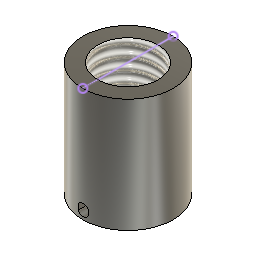
homemaderotoforgetoolholder v5 (Autodesk Fusion 360 archive; units mm, degrees)
design "homemaderotoforgetoolholder" references "autodesk 3ax table y head xz"
Autodesk Fusion 360 part; units mm, degrees
sketch "Sketch1" plane through (0, 0, 0) normal (0, 0, 1) x (1, 0, 0)
  circle A0 centre (0, 0) radius 3.175
  dimension "d1" = 6.35
  constraint coincident A0.centre origin
  measures "d1" diameter of A0
extrude "Extrude1" add sketch "Sketch1" along normal blind 8
sketch "Sketch2" plane through (0, 0, 8) normal (0, 0, 1) x (-1, 0, 0)
  circle A0 centre (0, 0) radius 3.175
  circle A1 centre (0, 0) radius 2
  constraint coincident A0.centre A1.centre
hole "Hole1" at (0, 0, 8) direction (0, 0, -1) diameter 4.234 depth 8 tip angle 180
thread "Thread1" "ISO Metric profile 5.0 M5x0.8 6H" major diameter 5.12 minor diameter 4.234 pitch 0.8 angle 60 resizes the face on face at (0.2108, -2.1065, 5.3333) from (0, 0, 8) to (0, 0, 1.5)
sketch "Sketch4" plane through (0, 0, 0) normal (1, 0, 0) x (0, 1, 0)
  line L0 (3.175, 8) -> (-3.175, 8)
sketch "Sketch5" plane through (0, 0, 0) normal (0, 0, -1) x (1, 0, 0)
  circle A0 centre (0, 0) radius 2.117
  circle A1 centre (0, 0) radius 3.175
  circle A2 centre (0, 0) radius 3.5
  circle A3 centre (0, 0) radius 2.117
  circle A4 centre (0, 0) radius 1.1
  dimension "d17" = 7
  dimension "d18" = 4.234
  dimension "d19" = 2.2
  constraint coincident A0.centre A1.centre
  constraint concentric A2 A3
  measures "d17" diameter of A2
  measures "d18" diameter of A3
  measures "d19" diameter of A4
extrude "Extrude3" add sketch "Sketch5" against normal blind 1.2 contours A0 A3
sketch "Sketch3" plane through (0, 0, 0) normal (0, 1, 0) x (1, 0, 0)
  line L0 (-0.5, -0.1) -> (0.5, -0.1)
  line L1 (0.5, -0.1) -> (0.5, -1.1)
  line L2 (0.5, -1.1) -> (-0.5, -1.1)
  line L3 (-0.5, -1.1) -> (-0.5, -0.1)
  line L4 (0, -1.75) -> (0, -22.5)
  line L5 (1.75, 0) -> (22.5, 0)
  circle A0 centre (0, -0.5996) radius 0.4064
  line L6 (0, -0.5996) -> (0, -1.1) construction
  line L7 (-0.35, -0.8061) -> (-0.35, -0.393)
  line L8 (0.35, -0.8061) -> (0.35, -0.393)
  dimension "d9" = 1
  dimension "d10" = 1
  dimension "d15" = 0.1
  dimension "d16" = 0.8128
  dimension "d24" = 0.4996
  dimension "d25" = 0.35
  constraint horizontal L0
  constraint vertical L1
  constraint horizontal L2
  constraint vertical L3
  constraint symmetric L1 L3 L4
  constraint coincident L4 A0.centre
  constraint midpoint L2 L6.end
  constraint perpendicular L2 L6
  constraint coincident A0.centre L6.start
  constraint coincident A0 L7.start
  constraint coincident A0 L7.end
  constraint parallel L3 L7
  constraint symmetric L6 L7.start L8.start
  constraint symmetric L6 L7.end L8.end
  measures "d9" distance of L0.start L0.end
  measures "d10" distance of L0.start L2.end
  measures "d15" distance of origin L0
  measures "d16" diameter of A0
  measures "d24" distance of L0 A0.centre
  measures "d25" distance of L6 L7
extrude "Extrude2" cut sketch "Sketch3" along normal mid plane 9 contours A0 L7 L8
fillet "Fillet2" [suppressed]
